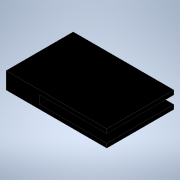
# Autodesk Inventor part: Flat Fastener
Saved by Autodesk Inventor 2020 (Build 240168000, 168)
## iProperties
Created: 2021-01-17
Part Number: Flat Fastener
Material: Generic
Document SubType Name: Modeling
Designer: magda
Density: 1 g/cm^3
Appearance: Default
Author: magda
Autodesk Inventor part; units mm, degrees
ref_plane "YZ Plane" through (0, 0, 0) normal (1, 0, 0) x (0, 1, 0)
ref_plane "XZ Plane" through (0, 0, 0) normal (0, 1, 0) x (-1, 0, 0)
ref_plane "XY Plane" through (0, 0, 0) normal (0, 0, 1) x (1, 0, 0)
sketch "Sketch1" plane through (0, 0, 0) normal (1, 0, 0) x (0, 1, 0)
  line L0 (1.3438, 16.5694) -> (-1.8312, 16.5694)
  line L1 (-1.8312, 16.5694) -> (-1.8312, -8.8306)
  line L2 (-1.8312, -8.8306) -> (1.3438, -8.8306)
  line L3 (1.3438, -8.8306) -> (1.3438, 16.5694)
  line L4 (1.3438, 16.5694) -> (2.9313, 16.5694)
  line L5 (2.9313, 16.5694) -> (2.9313, -8.8306)
  line L6 (2.9313, -8.8306) -> (1.3438, -8.8306)
  line L7 (1.3438, -8.8306) -> (1.3438, 16.5694)
  line L8 (-1.8312, 16.5694) -> (-3.4187, 16.5694)
  line L9 (-3.4187, 16.5694) -> (-3.4187, -8.8306)
  line L10 (-3.4187, -8.8306) -> (-1.8312, -8.8306)
  line L11 (-1.8312, -8.8306) -> (-1.8312, 16.5694)
  point P0 (0, 0)
  point P1 (-1.8312, -8.8306)
  point P2 (-1.8312, -8.8306)
  dimension "d0" = 3.175
  dimension "d1" = 25.4
  dimension "d2" = 1.5875
  dimension "d3" = 1.5875
  constraints: 24 end point, 6 parallel, 3 horizontal, 3 perpendicular, 1 point on line
  measures "d0" distance of L2.end L1.end
  measures "d1" distance of L0.end L1.end
  measures "d2" distance of L5.end L6.end
  measures "d3" distance of L10.end L9.end
extrude "Extrusion1" add sketch "Sketch1" along normal blind 25.4 contours L4 L5 L6 L3 | L1 L10 L9 L8
extrude "Extrusion2" add sketch "Sketch1" against normal blind 12.7
body "Solid1"
